Autodesk Fusion 360 part; units mm, degrees
(part 4 of 6)
sketch "Sketch5" plane through (0, 0, 0) normal (0, 1, 0) x (-1, 0, 0)
  arc A0 (-188.596, -16.7817) -> (-190.596, -18.7817) centre (-188.596, -18.7817) ccw
  line L0 (-190.596, -18.7817) -> (-190.596, -55.4069)
  line L1 (-190.596, -55.4069) -> (-190.59, -55.5639)
  line L2 (-190.59, -55.5639) -> (-190.572, -55.7209)
  line L3 (-190.572, -55.7209) -> (-190.54, -55.874)
  line L4 (-190.54, -55.874) -> (-190.499, -56.0268)
  line L5 (-190.499, -56.0268) -> (-190.444, -56.1728)
  line L6 (-190.444, -56.1728) -> (-190.379, -56.315)
  line L7 (-190.379, -56.315) -> (-190.302, -56.4526)
  line L8 (-190.302, -56.4526) -> (-190.215, -56.5838)
  line L9 (-190.215, -56.5838) -> (-190.117, -56.7062)
  line L10 (-190.117, -56.7062) -> (-190.011, -56.8219)
  line L11 (-190.011, -56.8219) -> (-189.895, -56.9281)
  line L12 (-189.895, -56.9281) -> (-189.771, -57.0258)
  line L13 (-189.771, -57.0258) -> (-189.64, -57.113)
  line L14 (-189.64, -57.113) -> (-189.504, -57.1899)
  line L15 (-189.504, -57.1899) -> (-189.362, -57.2548)
  line L16 (-189.362, -57.2548) -> (-189.214, -57.3098)
  line L17 (-189.214, -57.3098) -> (-189.063, -57.3525)
  line L18 (-189.063, -57.3525) -> (-188.908, -57.3828)
  line L19 (-188.908, -57.3828) -> (-188.753, -57.4008)
  line L20 (-188.753, -57.4008) -> (-188.597, -57.4075)
  line L21 (-188.597, -57.4075) -> (-184.1714, -57.4075)
  line L22 (-6.5216, -57.4075) -> (-2.096, -57.4075)
  line L23 (-2.096, -57.4075) -> (-1.9389, -57.4008)
  line L24 (-1.9389, -57.4008) -> (-1.7818, -57.3828)
  line L25 (-1.7818, -57.3828) -> (-1.6288, -57.3525)
  line L26 (-1.6288, -57.3525) -> (-1.4759, -57.3098)
  line L27 (-1.4759, -57.3098) -> (-1.3298, -57.2548)
  line L28 (-1.3298, -57.2548) -> (-1.1879, -57.1899)
  line L29 (-1.1879, -57.1899) -> (-1.0501, -57.113)
  line L30 (-1.0501, -57.113) -> (-0.9192, -57.0258)
  line L31 (-0.9192, -57.0258) -> (-0.7965, -56.9281)
  line L32 (-0.7965, -56.9281) -> (-0.6808, -56.8219)
  line L33 (-0.6808, -56.8219) -> (-0.5746, -56.7062)
  line L34 (-0.5746, -56.7062) -> (-0.4768, -56.5838)
  line L35 (-0.4768, -56.5838) -> (-0.39, -56.4526)
  line L36 (-0.39, -56.4526) -> (-0.3128, -56.315)
  line L37 (-0.3128, -56.315) -> (-0.248, -56.1728)
  line L38 (-0.248, -56.1728) -> (-0.1929, -56.0268)
  line L39 (-0.1929, -56.0268) -> (-0.1502, -55.874)
  line L40 (-0.1502, -55.874) -> (-0.1199, -55.7209)
  line L41 (-0.1199, -55.7209) -> (-0.102, -55.5639)
  line L42 (-0.102, -55.5639) -> (-0.0951, -55.4069)
  line L43 (-0.0951, -55.4069) -> (-0.0951, -18.7817)
  arc A1 (-0.0951, -18.7817) -> (-2.0951, -16.7817) centre (-2.0951, -18.7817) ccw
  line L44 (-2.0951, -16.7817) -> (-5.8454, -16.7817)
  arc A2 (-7.8454, -14.7817) -> (-5.8454, -16.7817) centre (-5.8454, -14.7817) ccw
  line L45 (-7.8454, -14.7817) -> (-7.8454, -2.2576)
  arc A3 (-7.8454, -2.2576) -> (-9.8454, -0.2576) centre (-9.8454, -2.2576) ccw
  line L46 (-9.8454, -0.2576) -> (-23.4739, -0.2575)
  arc A4 (-180.846, -0.2564) -> (-182.846, -2.2564) centre (-180.846, -2.2564) ccw
  line L47 (-182.846, -2.2564) -> (-182.846, -14.7817)
  arc A5 (-184.846, -16.7817) -> (-182.846, -14.7817) centre (-184.846, -14.7817) ccw
  line L48 (-184.846, -16.7817) -> (-188.596, -16.7817)
  line L49 (-31.196, -2.7823) -> (-31.196, -3.7827)
  line L50 (-31.196, -3.7827) -> (-30.3954, -3.7827)
  line L51 (-30.3954, -3.7827) -> (-30.3954, -6.8819)
  line L52 (-30.3954, -6.8819) -> (-31.196, -6.8819)
  line L53 (-31.196, -6.8819) -> (-31.196, -12.6821)
  line L54 (-31.196, -12.6821) -> (-30.3954, -12.6821)
  line L55 (-30.3954, -12.6821) -> (-30.3954, -15.7827)
  line L56 (-30.3954, -15.7827) -> (-31.196, -15.7827)
  line L57 (-31.196, -15.7827) -> (-31.196, -16.7817)
  line L58 (-31.196, -16.7817) -> (-45.1954, -16.7817)
  line L59 (-45.1954, -16.7817) -> (-45.1954, -15.7827)
  line L60 (-45.1954, -15.7827) -> (-45.9962, -15.7827)
  line L61 (-45.9962, -15.7827) -> (-45.9962, -12.6821)
  line L62 (-45.9962, -12.6821) -> (-45.1954, -12.6821)
  line L63 (-45.1954, -12.6821) -> (-45.1954, -6.8819)
  line L64 (-45.1954, -6.8819) -> (-45.9962, -6.8819)
  line L65 (-45.9962, -6.8819) -> (-45.9962, -3.7827)
  line L66 (-45.9962, -3.7827) -> (-45.1954, -3.7827)
  line L67 (-45.1954, -3.7827) -> (-45.1954, -2.7823)
  line L68 (-45.1954, -2.7823) -> (-31.196, -2.7823)
  line L69 (-159.495, -3.7827) -> (-159.495, -2.7823)
  line L70 (-159.495, -2.7823) -> (-145.496, -2.7823)
  line L71 (-145.496, -2.7823) -> (-145.496, -3.7827)
  line L72 (-145.496, -3.7827) -> (-144.695, -3.7827)
  line L73 (-144.695, -3.7827) -> (-144.695, -6.8819)
  line L74 (-144.695, -6.8819) -> (-145.496, -6.8819)
  line L75 (-145.496, -6.8819) -> (-145.496, -12.6821)
  line L76 (-145.496, -12.6821) -> (-144.695, -12.6821)
  line L77 (-144.695, -12.6821) -> (-144.695, -15.7827)
  line L78 (-144.695, -15.7827) -> (-145.496, -15.7827)
  line L79 (-145.496, -15.7827) -> (-145.496, -16.7817)
  line L80 (-145.496, -16.7817) -> (-159.495, -16.7817)
  line L81 (-159.495, -16.7817) -> (-159.495, -15.7827)
  line L82 (-159.495, -15.7827) -> (-160.296, -15.7827)
  line L83 (-160.296, -15.7827) -> (-160.296, -12.6821)
  line L84 (-160.296, -12.6821) -> (-159.495, -12.6821)
  line L85 (-159.495, -12.6821) -> (-159.495, -6.8819)
  line L86 (-159.495, -6.8819) -> (-160.296, -6.8819)
  line L87 (-160.296, -6.8819) -> (-160.296, -3.7827)
  line L88 (-160.296, -3.7827) -> (-159.495, -3.7827)
  line L89 (-59.7711, -40.8824) -> (-59.7711, -41.8828)
  line L90 (-59.7711, -41.8828) -> (-58.9703, -41.8828)
  line L91 (-58.9703, -41.8828) -> (-58.9703, -44.982)
  line L92 (-58.9703, -44.982) -> (-59.7711, -44.982)
  line L93 (-59.7711, -44.982) -> (-59.7711, -50.782)
  line L94 (-59.7711, -50.782) -> (-58.9703, -50.782)
  line L95 (-58.9703, -50.782) -> (-58.9703, -53.8826)
  line L96 (-58.9703, -53.8826) -> (-59.7711, -53.8826)
  line L97 (-59.7711, -53.8826) -> (-59.7711, -54.8816)
  line L98 (-59.7711, -54.8816) -> (-73.7704, -54.8816)
  line L99 (-73.7704, -54.8816) -> (-73.7704, -53.8826)
  line L100 (-73.7704, -53.8826) -> (-74.5712, -53.8826)
  line L101 (-74.5712, -53.8826) -> (-74.5712, -50.782)
  line L102 (-74.5712, -50.782) -> (-73.7704, -50.782)
  line L103 (-73.7704, -50.782) -> (-73.7704, -44.982)
  line L104 (-73.7704, -44.982) -> (-74.5712, -44.982)
  line L105 (-74.5712, -44.982) -> (-74.5712, -41.8828)
  line L106 (-74.5712, -41.8828) -> (-73.7704, -41.8828)
  line L107 (-73.7704, -41.8828) -> (-73.7704, -40.8824)
  line L108 (-73.7704, -40.8824) -> (-59.7711, -40.8824)
  line L109 (-92.8204, -54.8816) -> (-92.8204, -53.8826)
  line L110 (-92.8204, -53.8826) -> (-93.6198, -53.8826)
  line L111 (-93.6198, -53.8826) -> (-93.6198, -50.782)
  line L112 (-93.6198, -50.782) -> (-92.8204, -50.782)
  line L113 (-92.8204, -50.782) -> (-92.8204, -44.982)
  line L114 (-92.8204, -44.982) -> (-93.6198, -44.982)
  line L115 (-93.6198, -44.982) -> (-93.6198, -41.8828)
  line L116 (-93.6198, -41.8828) -> (-92.8204, -41.8828)
  line L117 (-92.8204, -41.8828) -> (-92.8204, -40.8824)
  line L118 (-92.8204, -40.8824) -> (-78.8211, -40.8824)
  line L119 (-78.8211, -40.8824) -> (-78.8211, -41.8828)
  line L120 (-78.8211, -41.8828) -> (-78.0203, -41.8828)
  line L121 (-78.0203, -41.8828) -> (-78.0203, -44.982)
  line L122 (-78.0203, -44.982) -> (-78.8211, -44.982)
  line L123 (-78.8211, -44.982) -> (-78.8211, -50.782)
  line L124 (-78.8211, -50.782) -> (-78.0203, -50.782)
  line L125 (-78.0203, -50.782) -> (-78.0203, -53.8826)
  line L126 (-78.0203, -53.8826) -> (-78.8211, -53.8826)
  line L127 (-78.8211, -53.8826) -> (-78.8211, -54.8816)
  line L128 (-78.8211, -54.8816) -> (-92.8204, -54.8816)
  line L129 (-16.6205, -54.8816) -> (-16.6205, -53.8826)
  line L130 (-16.6205, -53.8826) -> (-17.4212, -53.8826)
  line L131 (-17.4212, -53.8826) -> (-17.4212, -50.782)
  line L132 (-17.4212, -50.782) -> (-16.6205, -50.782)
  line L133 (-16.6205, -50.782) -> (-16.6205, -44.982)
  line L134 (-16.6205, -44.982) -> (-17.4212, -44.982)
  line L135 (-17.4212, -44.982) -> (-17.4212, -41.8828)
  line L136 (-17.4212, -41.8828) -> (-16.6205, -41.8828)
  line L137 (-16.6205, -41.8828) -> (-16.6205, -40.8824)
  line L138 (-16.6205, -40.8824) -> (-2.621, -40.8824)
  line L139 (-2.621, -40.8824) -> (-2.621, -41.8828)
  line L140 (-2.621, -41.8828) -> (-1.8204, -41.8828)
  line L141 (-1.8204, -41.8828) -> (-1.8204, -44.982)
  line L142 (-1.8204, -44.982) -> (-2.621, -44.982)
  line L143 (-2.621, -44.982) -> (-2.621, -50.782)
  line L144 (-2.621, -50.782) -> (-1.8204, -50.782)
  line L145 (-1.8204, -50.782) -> (-1.8204, -53.8826)
  line L146 (-1.8204, -53.8826) -> (-2.621, -53.8826)
  line L147 (-2.621, -53.8826) -> (-2.621, -54.8816)
  line L148 (-2.621, -54.8816) -> (-16.6205, -54.8816)
  line L149 (-174.071, -40.8824) -> (-174.071, -41.8828)
  line L150 (-174.071, -41.8828) -> (-173.27, -41.8828)
  line L151 (-173.27, -41.8828) -> (-173.27, -44.982)
  line L152 (-173.27, -44.982) -> (-174.071, -44.982)
  line L153 (-174.071, -44.982) -> (-174.071, -50.782)
  line L154 (-174.071, -50.782) -> (-173.27, -50.782)
  line L155 (-173.27, -50.782) -> (-173.27, -53.8826)
  line L156 (-173.27, -53.8826) -> (-174.071, -53.8826)
  line L157 (-174.071, -53.8826) -> (-174.071, -54.8816)
  line L158 (-174.071, -54.8816) -> (-188.07, -54.8816)
  line L159 (-188.07, -54.8816) -> (-188.07, -53.8826)
  line L160 (-188.07, -53.8826) -> (-188.871, -53.8826)
  line L161 (-188.871, -53.8826) -> (-188.871, -50.782)
  line L162 (-188.871, -50.782) -> (-188.07, -50.782)
  line L163 (-188.07, -50.782) -> (-188.07, -44.982)
  line L164 (-188.07, -44.982) -> (-188.871, -44.982)
  line L165 (-188.871, -44.982) -> (-188.871, -41.8828)
  line L166 (-188.871, -41.8828) -> (-188.07, -41.8828)
  line L167 (-188.07, -41.8828) -> (-188.07, -40.8824)
  line L168 (-188.07, -40.8824) -> (-174.071, -40.8824)
  line L169 (-126.446, -2.7823) -> (-126.446, -3.7827)
  line L170 (-126.446, -3.7827) -> (-125.645, -3.7827)
  line L171 (-125.645, -3.7827) -> (-125.645, -6.8819)
  line L172 (-125.645, -6.8819) -> (-126.446, -6.8819)
  line L173 (-126.446, -6.8819) -> (-126.446, -12.6821)
  line L174 (-126.446, -12.6821) -> (-125.645, -12.6821)
  line L175 (-125.645, -12.6821) -> (-125.645, -15.7827)
  line L176 (-125.645, -15.7827) -> (-126.446, -15.7827)
  line L177 (-126.446, -15.7827) -> (-126.446, -16.7817)
  line L178 (-126.446, -16.7817) -> (-140.445, -16.7817)
  line L179 (-140.445, -16.7817) -> (-140.445, -15.7827)
  line L180 (-140.445, -15.7827) -> (-141.246, -15.7827)
  line L181 (-141.246, -15.7827) -> (-141.246, -12.6821)
  line L182 (-141.246, -12.6821) -> (-140.445, -12.6821)
  line L183 (-140.445, -12.6821) -> (-140.445, -6.8819)
  line L184 (-140.445, -6.8819) -> (-141.246, -6.8819)
  line L185 (-141.246, -6.8819) -> (-141.246, -3.7827)
  line L186 (-141.246, -3.7827) -> (-140.445, -3.7827)
  line L187 (-140.445, -3.7827) -> (-140.445, -2.7823)
  line L188 (-140.445, -2.7823) -> (-126.446, -2.7823)
  line L189 (-26.1455, -16.7817) -> (-26.1455, -15.7827)
  line L190 (-26.1455, -15.7827) -> (-26.9462, -15.7827)
  line L191 (-26.9462, -15.7827) -> (-26.9462, -12.6821)
  line L192 (-26.9462, -12.6821) -> (-26.1455, -12.6821)
  line L193 (-26.1455, -12.6821) -> (-26.1455, -6.8819)
  line L194 (-26.1455, -6.8819) -> (-26.9462, -6.8819)
  line L195 (-26.9462, -6.8819) -> (-26.9462, -3.7827)
  line L196 (-26.9462, -3.7827) -> (-26.1455, -3.7827)
  line L197 (-26.1455, -3.7827) -> (-26.1455, -2.7823)
  line L198 (-26.1455, -2.7823) -> (-12.146, -2.7823)
  line L199 (-12.146, -2.7823) -> (-12.146, -3.7827)
  line L200 (-12.146, -3.7827) -> (-11.3454, -3.7827)
  line L201 (-11.3454, -3.7827) -> (-11.3454, -6.8819)
  line L202 (-11.3454, -6.8819) -> (-12.146, -6.8819)
  line L203 (-12.146, -6.8819) -> (-12.146, -12.6821)
  line L204 (-12.146, -12.6821) -> (-11.3454, -12.6821)
  line L205 (-11.3454, -12.6821) -> (-11.3454, -15.7827)
  line L206 (-11.3454, -15.7827) -> (-12.146, -15.7827)
  line L207 (-12.146, -15.7827) -> (-12.146, -16.7817)
  line L208 (-12.146, -16.7817) -> (-26.1455, -16.7817)
  line L209 (-64.2454, -3.7827) -> (-64.2454, -2.7823)
  line L210 (-64.2454, -2.7823) -> (-50.2461, -2.7823)
  line L211 (-50.2461, -2.7823) -> (-50.2461, -3.7827)
  line L212 (-50.2461, -3.7827) -> (-49.4453, -3.7827)
  line L213 (-49.4453, -3.7827) -> (-49.4453, -6.8819)
  line L214 (-49.4453, -6.8819) -> (-50.2461, -6.8819)
  line L215 (-50.2461, -6.8819) -> (-50.2461, -12.6821)
  line L216 (-50.2461, -12.6821) -> (-49.4453, -12.6821)
  line L217 (-49.4453, -12.6821) -> (-49.4453, -15.7827)
  line L218 (-49.4453, -15.7827) -> (-50.2461, -15.7827)
  line L219 (-50.2461, -15.7827) -> (-50.2461, -16.7817)
  line L220 (-50.2461, -16.7817) -> (-64.2454, -16.7817)
  line L221 (-64.2454, -16.7817) -> (-64.2454, -15.7827)
  line L222 (-64.2454, -15.7827) -> (-65.0462, -15.7827)
  line L223 (-65.0462, -15.7827) -> (-65.0462, -12.6821)
  line L224 (-65.0462, -12.6821) -> (-64.2454, -12.6821)
  line L225 (-64.2454, -12.6821) -> (-64.2454, -6.8819)
  line L226 (-64.2454, -6.8819) -> (-65.0462, -6.8819)
  line L227 (-65.0462, -6.8819) -> (-65.0462, -3.7827)
  line L228 (-65.0462, -3.7827) -> (-64.2454, -3.7827)
  line L229 (-135.971, -40.8824) -> (-135.971, -41.8828)
  line L230 (-135.971, -41.8828) -> (-135.17, -41.8828)
  line L231 (-135.17, -41.8828) -> (-135.17, -44.982)
  line L232 (-135.17, -44.982) -> (-135.971, -44.982)
  line L233 (-135.971, -44.982) -> (-135.971, -50.782)
  line L234 (-135.971, -50.782) -> (-135.17, -50.782)
  line L235 (-135.17, -50.782) -> (-135.17, -53.8826)
  line L236 (-135.17, -53.8826) -> (-135.971, -53.8826)
  line L237 (-135.971, -53.8826) -> (-135.971, -54.8816)
  line L238 (-135.971, -54.8816) -> (-149.97, -54.8816)
  line L239 (-149.97, -54.8816) -> (-149.97, -53.8826)
  line L240 (-149.97, -53.8826) -> (-150.771, -53.8826)
  line L241 (-150.771, -53.8826) -> (-150.771, -50.782)
  line L242 (-150.771, -50.782) -> (-149.97, -50.782)
  line L243 (-149.97, -50.782) -> (-149.97, -44.982)
  line L244 (-149.97, -44.982) -> (-150.771, -44.982)
  line L245 (-150.771, -44.982) -> (-150.771, -41.8828)
  line L246 (-150.771, -41.8828) -> (-149.97, -41.8828)
  line L247 (-149.97, -41.8828) -> (-149.97, -40.8824)
  line L248 (-149.97, -40.8824) -> (-135.971, -40.8824)
  line L249 (-73.7704, -35.8316) -> (-73.7704, -34.8327)
  line L250 (-73.7704, -34.8327) -> (-74.5712, -34.8327)
  line L251 (-74.5712, -34.8327) -> (-74.5712, -31.7321)
  line L252 (-74.5712, -31.7321) -> (-73.7704, -31.7321)
  line L253 (-73.7704, -31.7321) -> (-73.7704, -25.9319)
  line L254 (-73.7704, -25.9319) -> (-74.5712, -25.9319)
  line L255 (-74.5712, -25.9319) -> (-74.5712, -22.8327)
  line L256 (-74.5712, -22.8327) -> (-73.7704, -22.8327)
  line L257 (-73.7704, -22.8327) -> (-73.7704, -21.8323)
  line L258 (-73.7704, -21.8323) -> (-59.7711, -21.8323)
  line L259 (-59.7711, -21.8323) -> (-59.7711, -22.8327)
  line L260 (-59.7711, -22.8327) -> (-58.9703, -22.8327)
  line L261 (-58.9703, -22.8327) -> (-58.9703, -25.9319)
  line L262 (-58.9703, -25.9319) -> (-59.7711, -25.9319)
  line L263 (-59.7711, -25.9319) -> (-59.7711, -31.7321)
  line L264 (-59.7711, -31.7321) -> (-58.9703, -31.7321)
  line L265 (-58.9703, -31.7321) -> (-58.9703, -34.8327)
  line L266 (-58.9703, -34.8327) -> (-59.7711, -34.8327)
  line L267 (-59.7711, -34.8327) -> (-59.7711, -35.8316)
  line L268 (-59.7711, -35.8316) -> (-73.7704, -35.8316)
  line L269 (-54.7204, -41.8828) -> (-54.7204, -40.8824)
  line L270 (-54.7204, -40.8824) -> (-40.7211, -40.8824)
  line L271 (-40.7211, -40.8824) -> (-40.7211, -41.8828)
  line L272 (-40.7211, -41.8828) -> (-39.9203, -41.8828)
  line L273 (-39.9203, -41.8828) -> (-39.9203, -44.982)
  line L274 (-39.9203, -44.982) -> (-40.7211, -44.982)
  line L275 (-40.7211, -44.982) -> (-40.7211, -50.782)
  line L276 (-40.7211, -50.782) -> (-39.9203, -50.782)
  line L277 (-39.9203, -50.782) -> (-39.9203, -53.8826)
  line L278 (-39.9203, -53.8826) -> (-40.7211, -53.8826)
  line L279 (-40.7211, -53.8826) -> (-40.7211, -54.8816)
  line L280 (-40.7211, -54.8816) -> (-54.7204, -54.8816)
  line L281 (-54.7204, -54.8816) -> (-54.7204, -53.8826)
  line L282 (-54.7204, -53.8826) -> (-55.5212, -53.8826)
  line L283 (-55.5212, -53.8826) -> (-55.5212, -50.782)
  line L284 (-55.5212, -50.782) -> (-54.7204, -50.782)
  line L285 (-54.7204, -50.782) -> (-54.7204, -44.982)
  line L286 (-54.7204, -44.982) -> (-55.5212, -44.982)
  line L287 (-55.5212, -44.982) -> (-55.5212, -41.8828)
  line L288 (-55.5212, -41.8828) -> (-54.7204, -41.8828)
  line L289 (-130.92, -41.8828) -> (-130.92, -40.8824)
  line L290 (-130.92, -40.8824) -> (-116.92, -40.8824)
  line L291 (-116.92, -40.8824) -> (-116.92, -41.8828)
  line L292 (-116.92, -41.8828) -> (-116.119, -41.8828)
  line L293 (-116.119, -41.8828) -> (-116.119, -44.982)
  line L294 (-116.119, -44.982) -> (-116.92, -44.982)
  line L295 (-116.92, -44.982) -> (-116.92, -50.782)
  line L296 (-116.92, -50.782) -> (-116.119, -50.782)
  line L297 (-116.119, -50.782) -> (-116.119, -53.8826)
  line L298 (-116.119, -53.8826) -> (-116.92, -53.8826)
  line L299 (-116.92, -53.8826) -> (-116.92, -54.8816)
  line L300 (-116.92, -54.8816) -> (-130.92, -54.8816)
  line L301 (-130.92, -54.8816) -> (-130.92, -53.8826)
  line L302 (-130.92, -53.8826) -> (-131.721, -53.8826)
  line L303 (-131.721, -53.8826) -> (-131.721, -50.782)
  line L304 (-131.721, -50.782) -> (-130.92, -50.782)
  line L305 (-130.92, -50.782) -> (-130.92, -44.982)
  line L306 (-130.92, -44.982) -> (-131.721, -44.982)
  line L307 (-131.721, -44.982) -> (-131.721, -41.8828)
  line L308 (-131.721, -41.8828) -> (-130.92, -41.8828)
  line L309 (-21.671, -53.8826) -> (-21.671, -54.8816)
  line L310 (-21.671, -54.8816) -> (-35.6704, -54.8816)
  line L311 (-35.6704, -54.8816) -> (-35.6704, -53.8826)
  line L312 (-35.6704, -53.8826) -> (-36.4712, -53.8826)
  line L313 (-36.4712, -53.8826) -> (-36.4712, -50.782)
  line L314 (-36.4712, -50.782) -> (-35.6704, -50.782)
  line L315 (-35.6704, -50.782) -> (-35.6704, -44.982)
  line L316 (-35.6704, -44.982) -> (-36.4712, -44.982)
  line L317 (-36.4712, -44.982) -> (-36.4712, -41.8828)
  line L318 (-36.4712, -41.8828) -> (-35.6704, -41.8828)
  line L319 (-35.6704, -41.8828) -> (-35.6704, -40.8824)
  line L320 (-35.6704, -40.8824) -> (-21.671, -40.8824)
  line L321 (-21.671, -40.8824) -> (-21.671, -41.8828)
  line L322 (-21.671, -41.8828) -> (-20.8704, -41.8828)
  line L323 (-20.8704, -41.8828) -> (-20.8704, -44.982)
  line L324 (-20.8704, -44.982) -> (-21.671, -44.982)
  line L325 (-21.671, -44.982) -> (-21.671, -50.782)
  line L326 (-21.671, -50.782) -> (-20.8704, -50.782)
  line L327 (-20.8704, -50.782) -> (-20.8704, -53.8826)
  line L328 (-20.8704, -53.8826) -> (-21.671, -53.8826)
  line L329 (-97.8697, -53.8826) -> (-97.8697, -54.8816)
  line L330 (-97.8697, -54.8816) -> (-111.869, -54.8816)
  line L331 (-111.869, -54.8816) -> (-111.869, -53.8826)
  line L332 (-111.869, -53.8826) -> (-112.67, -53.8826)
  line L333 (-112.67, -53.8826) -> (-112.67, -50.782)
  line L334 (-112.67, -50.782) -> (-111.869, -50.782)
  line L335 (-111.869, -50.782) -> (-111.869, -44.982)
  line L336 (-111.869, -44.982) -> (-112.67, -44.982)
  line L337 (-112.67, -44.982) -> (-112.67, -41.8828)
  line L338 (-112.67, -41.8828) -> (-111.869, -41.8828)
  line L339 (-111.869, -41.8828) -> (-111.869, -40.8824)
  line L340 (-111.869, -40.8824) -> (-97.8697, -40.8824)
  line L341 (-97.8697, -40.8824) -> (-97.8697, -41.8828)
  line L342 (-97.8697, -41.8828) -> (-97.0703, -41.8828)
  line L343 (-97.0703, -41.8828) -> (-97.0703, -44.982)
  line L344 (-97.0703, -44.982) -> (-97.8697, -44.982)
  line L345 (-97.8697, -44.982) -> (-97.8697, -50.782)
  line L346 (-97.8697, -50.782) -> (-97.0703, -50.782)
  line L347 (-97.0703, -50.782) -> (-97.0703, -53.8826)
  line L348 (-97.0703, -53.8826) -> (-97.8697, -53.8826)
  line L349 (-155.021, -53.8826) -> (-155.021, -54.8816)
  line L350 (-155.021, -54.8816) -> (-169.02, -54.8816)
  line L351 (-169.02, -54.8816) -> (-169.02, -53.8826)
  line L352 (-169.02, -53.8826) -> (-169.821, -53.8826)
  line L353 (-169.821, -53.8826) -> (-169.821, -50.782)
  line L354 (-169.821, -50.782) -> (-169.02, -50.782)
  line L355 (-169.02, -50.782) -> (-169.02, -44.982)
  line L356 (-169.02, -44.982) -> (-169.821, -44.982)
  line L357 (-169.821, -44.982) -> (-169.821, -41.8828)
  line L358 (-169.821, -41.8828) -> (-169.02, -41.8828)
  line L359 (-169.02, -41.8828) -> (-169.02, -40.8824)
  line L360 (-169.02, -40.8824) -> (-155.021, -40.8824)
  line L361 (-155.021, -40.8824) -> (-155.021, -41.8828)
  line L362 (-155.021, -41.8828) -> (-154.22, -41.8828)
  line L363 (-154.22, -41.8828) -> (-154.22, -44.982)
  line L364 (-154.22, -44.982) -> (-155.021, -44.982)
  line L365 (-155.021, -44.982) -> (-155.021, -50.782)
  line L366 (-155.021, -50.782) -> (-154.22, -50.782)
  line L367 (-154.22, -50.782) -> (-154.22, -53.8826)
  line L368 (-154.22, -53.8826) -> (-155.021, -53.8826)
  line L369 (-111.87, -16.7817) -> (-111.87, -15.7827)
  line L370 (-111.87, -15.7827) -> (-112.671, -15.7827)
  line L371 (-112.671, -15.7827) -> (-112.671, -12.6821)
  line L372 (-112.671, -12.6821) -> (-111.87, -12.6821)
  line L373 (-111.87, -12.6821) -> (-111.87, -12.0826)
  line L374 (-111.87, -12.0826) -> (-113.396, -12.0826)
  line L375 (-113.396, -12.0826) -> (-113.396, -15.3128)
  line L376 (-113.396, -15.3128) -> (-115.12, -15.3128)
  line L377 (-115.12, -15.3128) -> (-115.12, -16.2319)
  line L378 (-115.12, -16.2319) -> (-118.42, -16.2319)
  line L379 (-118.42, -16.2319) -> (-118.42, -15.3128)
  line L380 (-118.42, -15.3128) -> (-120.146, -15.3128)
  line L381 (-120.146, -15.3128) -> (-120.146, -12.0826)
  line L382 (-120.146, -12.0826) -> (-120.971, -12.0826)
  line L383 (-120.971, -12.0826) -> (-120.971, -9.2825)
  line L384 (-120.971, -9.2825) -> (-120.146, -9.2825)
  line L385 (-120.146, -9.2825) -> (-120.146, -3.0138)
  line L386 (-120.146, -3.0138) -> (-118.42, -3.0138)
  line L387 (-118.42, -3.0138) -> (-118.42, -2.0326)
  line L388 (-118.42, -2.0326) -> (-115.12, -2.0326)
  line L389 (-115.12, -2.0326) -> (-115.12, -3.0138)
  line L390 (-115.12, -3.0138) -> (-113.396, -3.0138)
  line L391 (-113.396, -3.0138) -> (-113.396, -7.4827)
  line L392 (-113.396, -7.4827) -> (-111.87, -7.4827)
  line L393 (-111.87, -7.4827) -> (-111.87, -6.8819)
  line L394 (-111.87, -6.8819) -> (-112.671, -6.8819)
  line L395 (-112.671, -6.8819) -> (-112.671, -3.7827)
  line L396 (-112.671, -3.7827) -> (-111.87, -3.7827)
  line L397 (-111.87, -3.7827) -> (-111.87, -2.7823)
  line L398 (-111.87, -2.7823) -> (-97.8711, -2.7823)
  line L399 (-97.8711, -2.7823) -> (-97.8711, -3.7827)
  line L400 (-97.8711, -3.7827) -> (-97.0703, -3.7827)
  line L401 (-97.0703, -3.7827) -> (-97.0703, -6.8819)
  line L402 (-97.0703, -6.8819) -> (-97.8711, -6.8819)
  line L403 (-97.8711, -6.8819) -> (-97.8711, -7.4827)
  line L404 (-97.8711, -7.4827) -> (-96.3454, -7.4827)
  line L405 (-96.3454, -7.4827) -> (-96.3454, -3.0138)
  line L406 (-96.3454, -3.0138) -> (-94.6203, -3.0138)
  line L407 (-94.6203, -3.0138) -> (-94.6203, -2.0326)
  line L408 (-94.6203, -2.0326) -> (-91.3197, -2.0326)
  line L409 (-91.3197, -2.0326) -> (-91.3197, -3.0138)
  line L410 (-91.3197, -3.0138) -> (-89.596, -3.0138)
  line L411 (-89.596, -3.0138) -> (-89.596, -9.2825)
  line L412 (-89.596, -9.2825) -> (-88.7705, -9.2825)
  line L413 (-88.7705, -9.2825) -> (-88.7705, -12.0826)
  line L414 (-88.7705, -12.0826) -> (-89.596, -12.0826)
  line L415 (-89.596, -12.0826) -> (-89.596, -15.3128)
  line L416 (-89.596, -15.3128) -> (-91.3197, -15.3128)
  line L417 (-91.3197, -15.3128) -> (-91.3197, -16.2319)
  line L418 (-91.3197, -16.2319) -> (-94.6203, -16.2319)
  line L419 (-94.6203, -16.2319) -> (-94.6203, -15.3128)
  line L420 (-94.6203, -15.3128) -> (-96.3454, -15.3128)
  line L421 (-96.3454, -15.3128) -> (-96.3454, -12.0826)
  line L422 (-96.3454, -12.0826) -> (-97.8711, -12.0826)
  line L423 (-97.8711, -12.0826) -> (-97.8711, -12.6821)
  line L424 (-97.8711, -12.6821) -> (-97.0703, -12.6821)
  line L425 (-97.0703, -12.6821) -> (-97.0703, -15.7827)
  line L426 (-97.0703, -15.7827) -> (-97.8711, -15.7827)
  line L427 (-97.8711, -15.7827) -> (-97.8711, -16.7817)
  line L428 (-97.8711, -16.7817) -> (-111.87, -16.7817)
  line L429 (-69.2961, -15.7827) -> (-69.2961, -16.7817)
  line L430 (-69.2961, -16.7817) -> (-83.2954, -16.7817)
  line L431 (-83.2954, -16.7817) -> (-83.2954, -15.7827)
  line L432 (-83.2954, -15.7827) -> (-84.0962, -15.7827)
  line L433 (-84.0962, -15.7827) -> (-84.0962, -12.6821)
  line L434 (-84.0962, -12.6821) -> (-83.2954, -12.6821)
  line L435 (-83.2954, -12.6821) -> (-83.2954, -6.8819)
  line L436 (-83.2954, -6.8819) -> (-84.0962, -6.8819)
  line L437 (-84.0962, -6.8819) -> (-84.0962, -3.7827)
  line L438 (-84.0962, -3.7827) -> (-83.2954, -3.7827)
  line L439 (-83.2954, -3.7827) -> (-83.2954, -2.7823)
  line L440 (-83.2954, -2.7823) -> (-69.2961, -2.7823)
  line L441 (-69.2961, -2.7823) -> (-69.2961, -3.7827)
  line L442 (-69.2961, -3.7827) -> (-68.4953, -3.7827)
  line L443 (-68.4953, -3.7827) -> (-68.4953, -6.8819)
  line L444 (-68.4953, -6.8819) -> (-69.2961, -6.8819)
  line L445 (-69.2961, -6.8819) -> (-69.2961, -12.6821)
  line L446 (-69.2961, -12.6821) -> (-68.4953, -12.6821)
  line L447 (-68.4953, -12.6821) -> (-68.4953, -15.7827)
  line L448 (-68.4953, -15.7827) -> (-69.2961, -15.7827)
  line L449 (-40.7211, -34.8327) -> (-40.7211, -35.8316)
  line L450 (-40.7211, -35.8316) -> (-54.7204, -35.8316)
  line L451 (-54.7204, -35.8316) -> (-54.7204, -34.8327)
  line L452 (-54.7204, -34.8327) -> (-55.5212, -34.8327)
  line L453 (-55.5212, -34.8327) -> (-55.5212, -31.7321)
  line L454 (-55.5212, -31.7321) -> (-54.7204, -31.7321)
  line L455 (-54.7204, -31.7321) -> (-54.7204, -25.9319)
  line L456 (-54.7204, -25.9319) -> (-55.5212, -25.9319)
  line L457 (-55.5212, -25.9319) -> (-55.5212, -22.8327)
  line L458 (-55.5212, -22.8327) -> (-54.7204, -22.8327)
  line L459 (-54.7204, -22.8327) -> (-54.7204, -21.8323)
  line L460 (-54.7204, -21.8323) -> (-40.7211, -21.8323)
  line L461 (-40.7211, -21.8323) -> (-40.7211, -22.8327)
  line L462 (-40.7211, -22.8327) -> (-39.9203, -22.8327)
  line L463 (-39.9203, -22.8327) -> (-39.9203, -25.9319)
  line L464 (-39.9203, -25.9319) -> (-40.7211, -25.9319)
  line L465 (-40.7211, -25.9319) -> (-40.7211, -31.7321)
  line L466 (-40.7211, -31.7321) -> (-39.9203, -31.7321)
  line L467 (-39.9203, -31.7321) -> (-39.9203, -34.8327)
  line L468 (-39.9203, -34.8327) -> (-40.7211, -34.8327)
  line L469 (-111.869, -22.8327) -> (-111.869, -21.8323)
  line L470 (-111.869, -21.8323) -> (-97.8697, -21.8323)
  line L471 (-97.8697, -21.8323) -> (-97.8697, -22.8327)
  line L472 (-97.8697, -22.8327) -> (-97.0703, -22.8327)
  line L473 (-97.0703, -22.8327) -> (-97.0703, -25.9319)
  line L474 (-97.0703, -25.9319) -> (-97.8697, -25.9319)
  line L475 (-97.8697, -25.9319) -> (-97.8697, -31.7321)
  line L476 (-97.8697, -31.7321) -> (-97.0703, -31.7321)
  line L477 (-97.0703, -31.7321) -> (-97.0703, -34.8327)
  line L478 (-97.0703, -34.8327) -> (-97.8697, -34.8327)
  line L479 (-97.8697, -34.8327) -> (-97.8697, -35.8316)
  line L480 (-97.8697, -35.8316) -> (-111.869, -35.8316)
  line L481 (-111.869, -35.8316) -> (-111.869, -34.8327)
  line L482 (-111.869, -34.8327) -> (-112.67, -34.8327)
  line L483 (-112.67, -34.8327) -> (-112.67, -31.7321)
  line L484 (-112.67, -31.7321) -> (-111.869, -31.7321)
  line L485 (-111.869, -31.7321) -> (-111.869, -25.9319)
  line L486 (-111.869, -25.9319) -> (-112.67, -25.9319)
  line L487 (-112.67, -25.9319) -> (-112.67, -22.8327)
  line L488 (-112.67, -22.8327) -> (-111.869, -22.8327)
  line L489 (-92.8204, -22.8327) -> (-92.8204, -21.8323)
  line L490 (-92.8204, -21.8323) -> (-78.8211, -21.8323)
  line L491 (-78.8211, -21.8323) -> (-78.8211, -22.8327)
  line L492 (-78.8211, -22.8327) -> (-78.0203, -22.8327)
  line L493 (-78.0203, -22.8327) -> (-78.0203, -25.9319)
  line L494 (-78.0203, -25.9319) -> (-78.8211, -25.9319)
  line L495 (-78.8211, -25.9319) -> (-78.8211, -31.7321)
  line L496 (-78.8211, -31.7321) -> (-78.0203, -31.7321)
  line L497 (-78.0203, -31.7321) -> (-78.0203, -34.8327)
  line L498 (-78.0203, -34.8327) -> (-78.8211, -34.8327)
  line L499 (-78.8211, -34.8327) -> (-78.8211, -35.8316)
  line L500 (-78.8211, -35.8316) -> (-92.8204, -35.8316)
  line L501 (-92.8204, -35.8316) -> (-92.8204, -34.8327)
  line L502 (-92.8204, -34.8327) -> (-93.6198, -34.8327)
  line L503 (-93.6198, -34.8327) -> (-93.6198, -31.7321)
  line L504 (-93.6198, -31.7321) -> (-92.8204, -31.7321)
  line L505 (-92.8204, -31.7321) -> (-92.8204, -25.9319)
  line L506 (-92.8204, -25.9319) -> (-93.6198, -25.9319)
  line L507 (-93.6198, -25.9319) -> (-93.6198, -22.8327)
  line L508 (-93.6198, -22.8327) -> (-92.8204, -22.8327)
  line L509 (-35.6704, -22.8327) -> (-35.6704, -21.8323)
  line L510 (-35.6704, -21.8323) -> (-21.671, -21.8323)
  line L511 (-21.671, -21.8323) -> (-21.671, -22.8327)
  line L512 (-21.671, -22.8327) -> (-20.8704, -22.8327)
  line L513 (-20.8704, -22.8327) -> (-20.8704, -25.9319)
  line L514 (-20.8704, -25.9319) -> (-21.671, -25.9319)
  line L515 (-21.671, -25.9319) -> (-21.671, -31.7321)
  line L516 (-21.671, -31.7321) -> (-20.8704, -31.7321)
  line L517 (-20.8704, -31.7321) -> (-20.8704, -34.8327)
  line L518 (-20.8704, -34.8327) -> (-21.671, -34.8327)
  line L519 (-21.671, -34.8327) -> (-21.671, -35.8316)
  line L520 (-21.671, -35.8316) -> (-35.6704, -35.8316)
  line L521 (-35.6704, -35.8316) -> (-35.6704, -34.8327)
  line L522 (-35.6704, -34.8327) -> (-36.4712, -34.8327)
  line L523 (-36.4712, -34.8327) -> (-36.4712, -31.7321)
  line L524 (-36.4712, -31.7321) -> (-35.6704, -31.7321)
  line L525 (-35.6704, -31.7321) -> (-35.6704, -25.9319)
  line L526 (-35.6704, -25.9319) -> (-36.4712, -25.9319)
  line L527 (-36.4712, -25.9319) -> (-36.4712, -22.8327)
  line L528 (-36.4712, -22.8327) -> (-35.6704, -22.8327)
  line L529 (-16.6205, -22.8327) -> (-16.6205, -21.8323)
  line L530 (-16.6205, -21.8323) -> (-2.621, -21.8323)
  line L531 (-2.621, -21.8323) -> (-2.621, -22.8327)
  line L532 (-2.621, -22.8327) -> (-1.8204, -22.8327)
  line L533 (-1.8204, -22.8327) -> (-1.8204, -25.9319)
  line L534 (-1.8204, -25.9319) -> (-2.621, -25.9319)
  line L535 (-2.621, -25.9319) -> (-2.621, -31.7321)
  line L536 (-2.621, -31.7321) -> (-1.8204, -31.7321)
  line L537 (-1.8204, -31.7321) -> (-1.8204, -34.8327)
  line L538 (-1.8204, -34.8327) -> (-2.621, -34.8327)
  line L539 (-2.621, -34.8327) -> (-2.621, -35.8316)
  line L540 (-2.621, -35.8316) -> (-16.6205, -35.8316)
  line L541 (-16.6205, -35.8316) -> (-16.6205, -34.8327)
  line L542 (-16.6205, -34.8327) -> (-17.4212, -34.8327)
  line L543 (-17.4212, -34.8327) -> (-17.4212, -31.7321)
  line L544 (-17.4212, -31.7321) -> (-16.6205, -31.7321)
  line L545 (-16.6205, -31.7321) -> (-16.6205, -25.9319)
  line L546 (-16.6205, -25.9319) -> (-17.4212, -25.9319)
  line L547 (-17.4212, -25.9319) -> (-17.4212, -22.8327)
  line L548 (-17.4212, -22.8327) -> (-16.6205, -22.8327)
  line L549 (-164.546, -15.7827) -> (-164.546, -16.7817)
  line L550 (-164.546, -16.7817) -> (-178.545, -16.7817)
  line L551 (-178.545, -16.7817) -> (-178.545, -15.7827)
  line L552 (-178.545, -15.7827) -> (-179.346, -15.7827)
  line L553 (-179.346, -15.7827) -> (-179.346, -12.6821)
  line L554 (-179.346, -12.6821) -> (-178.545, -12.6821)
  line L555 (-178.545, -12.6821) -> (-178.545, -6.8819)
  line L556 (-178.545, -6.8819) -> (-179.346, -6.8819)
  line L557 (-179.346, -6.8819) -> (-179.346, -3.7827)
  line L558 (-179.346, -3.7827) -> (-178.545, -3.7827)
  line L559 (-178.545, -3.7827) -> (-178.545, -2.7823)
  line L560 (-178.545, -2.7823) -> (-164.546, -2.7823)
  line L561 (-164.546, -2.7823) -> (-164.546, -3.7827)
  line L562 (-164.546, -3.7827) -> (-163.745, -3.7827)
  line L563 (-163.745, -3.7827) -> (-163.745, -6.8819)
  line L564 (-163.745, -6.8819) -> (-164.546, -6.8819)
  line L565 (-164.546, -6.8819) -> (-164.546, -12.6821)
  line L566 (-164.546, -12.6821) -> (-163.745, -12.6821)
  line L567 (-163.745, -12.6821) -> (-163.745, -15.7827)
  line L568 (-163.745, -15.7827) -> (-164.546, -15.7827)
  line L569 (-116.92, -34.8327) -> (-116.92, -35.8316)
  line L570 (-116.92, -35.8316) -> (-130.92, -35.8316)
  line L571 (-130.92, -35.8316) -> (-130.92, -34.8327)
  line L572 (-130.92, -34.8327) -> (-131.721, -34.8327)
  line L573 (-131.721, -34.8327) -> (-131.721, -31.7321)
  line L574 (-131.721, -31.7321) -> (-130.92, -31.7321)
  line L575 (-130.92, -31.7321) -> (-130.92, -25.9319)
  line L576 (-130.92, -25.9319) -> (-131.721, -25.9319)
  line L577 (-131.721, -25.9319) -> (-131.721, -22.8327)
  line L578 (-131.721, -22.8327) -> (-130.92, -22.8327)
  line L579 (-130.92, -22.8327) -> (-130.92, -21.8323)
  line L580 (-130.92, -21.8323) -> (-116.92, -21.8323)
  line L581 (-116.92, -21.8323) -> (-116.92, -22.8327)
  line L582 (-116.92, -22.8327) -> (-116.119, -22.8327)
  line L583 (-116.119, -22.8327) -> (-116.119, -25.9319)
  line L584 (-116.119, -25.9319) -> (-116.92, -25.9319)
  line L585 (-116.92, -25.9319) -> (-116.92, -31.7321)
  line L586 (-116.92, -31.7321) -> (-116.119, -31.7321)
  line L587 (-116.119, -31.7321) -> (-116.119, -34.8327)
  line L588 (-116.119, -34.8327) -> (-116.92, -34.8327)
  line L589 (-155.021, -34.8327) -> (-155.021, -35.8316)
  line L590 (-155.021, -35.8316) -> (-169.02, -35.8316)
  line L591 (-169.02, -35.8316) -> (-169.02, -34.8327)
  line L592 (-169.02, -34.8327) -> (-169.821, -34.8327)
  line L593 (-169.821, -34.8327) -> (-169.821, -31.7321)
  line L594 (-169.821, -31.7321) -> (-169.02, -31.7321)
  line L595 (-169.02, -31.7321) -> (-169.02, -25.9319)
  line L596 (-169.02, -25.9319) -> (-169.821, -25.9319)
  line L597 (-169.821, -25.9319) -> (-169.821, -22.8327)
  line L598 (-169.821, -22.8327) -> (-169.02, -22.8327)
  line L599 (-169.02, -22.8327) -> (-169.02, -21.8323)
  line L600 (-169.02, -21.8323) -> (-155.021, -21.8323)
  line L601 (-155.021, -21.8323) -> (-155.021, -22.8327)
  line L602 (-155.021, -22.8327) -> (-154.22, -22.8327)
  line L603 (-154.22, -22.8327) -> (-154.22, -25.9319)
  line L604 (-154.22, -25.9319) -> (-155.021, -25.9319)
  line L605 (-155.021, -25.9319) -> (-155.021, -31.7321)
  line L606 (-155.021, -31.7321) -> (-154.22, -31.7321)
  line L607 (-154.22, -31.7321) -> (-154.22, -34.8327)
  line L608 (-154.22, -34.8327) -> (-155.021, -34.8327)
  line L609 (-135.971, -34.8327) -> (-135.971, -35.8316)
  line L610 (-135.971, -35.8316) -> (-149.97, -35.8316)
  line L611 (-149.97, -35.8316) -> (-149.97, -34.8327)
  line L612 (-149.97, -34.8327) -> (-150.771, -34.8327)
  line L613 (-150.771, -34.8327) -> (-150.771, -31.7321)
  line L614 (-150.771, -31.7321) -> (-149.97, -31.7321)
  line L615 (-149.97, -31.7321) -> (-149.97, -25.9319)
  line L616 (-149.97, -25.9319) -> (-150.771, -25.9319)
  line L617 (-150.771, -25.9319) -> (-150.771, -22.8327)
  line L618 (-150.771, -22.8327) -> (-149.97, -22.8327)
  line L619 (-149.97, -22.8327) -> (-149.97, -21.8323)
  line L620 (-149.97, -21.8323) -> (-135.971, -21.8323)
  line L621 (-135.971, -21.8323) -> (-135.971, -22.8327)
  line L622 (-135.971, -22.8327) -> (-135.17, -22.8327)
  line L623 (-135.17, -22.8327) -> (-135.17, -25.9319)
  line L624 (-135.17, -25.9319) -> (-135.971, -25.9319)
  line L625 (-135.971, -25.9319) -> (-135.971, -31.7321)
  line L626 (-135.971, -31.7321) -> (-135.17, -31.7321)
  line L627 (-135.17, -31.7321) -> (-135.17, -34.8327)
  line L628 (-135.17, -34.8327) -> (-135.971, -34.8327)
  line L629 (-188.07, -22.8327) -> (-188.07, -21.8323)
  line L630 (-188.07, -21.8323) -> (-174.071, -21.8323)
  line L631 (-174.071, -21.8323) -> (-174.071, -22.8327)
  line L632 (-174.071, -22.8327) -> (-173.27, -22.8327)
  line L633 (-173.27, -22.8327) -> (-173.27, -25.9319)
  line L634 (-173.27, -25.9319) -> (-174.071, -25.9319)
  line L635 (-174.071, -25.9319) -> (-174.071, -31.7321)
  line L636 (-174.071, -31.7321) -> (-173.27, -31.7321)
  line L637 (-173.27, -31.7321) -> (-173.27, -34.8327)
  line L638 (-173.27, -34.8327) -> (-174.071, -34.8327)
  line L639 (-174.071, -34.8327) -> (-174.071, -35.8316)
  line L640 (-174.071, -35.8316) -> (-188.07, -35.8316)
  line L641 (-188.07, -35.8316) -> (-188.07, -34.8327)
  line L642 (-188.07, -34.8327) -> (-188.871, -34.8327)
  line L643 (-188.871, -34.8327) -> (-188.871, -31.7321)
  line L644 (-188.871, -31.7321) -> (-188.07, -31.7321)
  line L645 (-188.07, -31.7321) -> (-188.07, -25.9319)
  line L646 (-188.07, -25.9319) -> (-188.871, -25.9319)
  line L647 (-188.871, -25.9319) -> (-188.871, -22.8327)
  line L648 (-188.871, -22.8327) -> (-188.07, -22.8327)
  line L649 (-118.42, -2.0326) -> (-120.971, -2.0326)
  line L650 (-120.971, -2.0326) -> (-120.971, -12.0826)
  line L651 (-88.7705, -16.7817) -> (-120.971, -16.7817)
  line L652 (-120.971, -16.7817) -> (-120.971, -2.0326)
  line L653 (-120.971, -2.0326) -> (-88.7705, -2.0326)
  line L654 (-88.7705, -2.0326) -> (-88.7705, -16.7817)
  spline S0 degree 2 poles (-184.1714, -57.4075) (-176.3801, -57.4075) (-176.3801, -64.9763) knots 0 0 0 1 1 1
  arc A6 (-176.3801, -64.9763) -> (-162.7837, -64.9763) centre (-169.5819, -64.5335) ccw
  spline S1 degree 2 poles (-154.9924, -57.4075) (-162.7837, -57.4075) (-162.7837, -64.9763) knots 0 0 0 1 1 1
  line L655 (-154.9924, -57.4075) -> (-35.7006, -57.4075)
  spline S2 degree 2 poles (-35.7006, -57.4075) (-27.9093, -57.4075) (-27.9093, -64.9763) knots 0 0 0 1 1 1
  arc A7 (-27.9093, -64.9763) -> (-14.3129, -64.9763) centre (-21.1111, -64.5335) ccw
  spline S3 degree 2 poles (-6.5216, -57.4075) (-14.3129, -57.4075) (-14.3129, -64.9763) knots 0 0 0 1 1 1
  line L656 (-167.2132, -68.8727) -> (-171.8315, -68.9414)
  line L657 (-171.8315, -68.9414) -> (-174.2002, -64.9763)
  line L658 (-174.2002, -64.9763) -> (-171.9506, -60.9423)
  line L659 (-171.9506, -60.9423) -> (-167.3323, -60.8736)
  line L660 (-167.3323, -60.8736) -> (-164.9636, -64.8387)
  line L661 (-164.9636, -64.8387) -> (-167.2132, -68.8727)
  line L662 (-18.8615, -68.9414) -> (-23.4798, -68.8727)
  line L663 (-23.4798, -68.8727) -> (-25.7294, -64.8387)
  line L664 (-25.7294, -64.8387) -> (-23.3607, -60.8736)
  line L665 (-23.3607, -60.8736) -> (-18.7424, -60.9423)
  line L666 (-18.7424, -60.9423) -> (-16.4928, -64.9763)
  line L667 (-16.4928, -64.9763) -> (-18.8615, -68.9414)
  spline S4 degree 2 poles (-23.4739, -0.2575) (-31.3819, -0.2565) (-31.3817, 7.3119) knots 0 0 0 1 1 1
  arc A8 (-31.3817, 7.3119) -> (-44.977, 7.3123) centre (-38.1793, 6.8699) ccw
  spline S5 degree 2 poles (-52.8852, -0.2567) (-44.9772, -0.2561) (-44.977, 7.3123) knots 0 0 0 1 1 1
  line L668 (-52.8852, -0.2567) -> (-52.887, -0.2573)
  line L669 (-52.887, -0.2573) -> (-137.8078, -0.2567)
  spline S6 degree 2 poles (-137.8078, -0.2567) (-145.7158, -0.2561) (-145.716, 7.3123) knots 0 0 0 1 1 1
  arc A9 (-145.716, 7.3123) -> (-159.3113, 7.3119) centre (-152.5137, 6.8699) ccw
  spline S7 degree 2 poles (-167.0351, -0.2565) (-159.3111, -0.1679) (-159.3113, 7.3119) knots 0.011703 0.011703 0.011703 1 1 1
  line L670 (-167.0351, -0.2565) -> (-180.846, -0.2564)
  line L671 (-35.9298, 3.2095) -> (-40.548, 3.2783)
  line L672 (-40.548, 3.2783) -> (-42.7976, 7.3122)
  line L673 (-42.7976, 7.3122) -> (-40.4289, 11.2774)
  line L674 (-40.4289, 11.2774) -> (-35.8106, 11.2086)
  line L675 (-35.8106, 11.2086) -> (-33.561, 7.1747)
  line L676 (-33.561, 7.1747) -> (-35.9298, 3.2095)
  line L677 (-154.7632, 3.2095) -> (-157.132, 7.1747)
  line L678 (-157.132, 7.1747) -> (-154.8824, 11.2086)
  line L679 (-154.8824, 11.2086) -> (-150.2641, 11.2774)
  line L680 (-150.2641, 11.2774) -> (-147.8954, 7.3122)
  line L681 (-147.8954, 7.3122) -> (-150.145, 3.2783)
  line L682 (-150.145, 3.2783) -> (-154.7632, 3.2095)
  point P0 (-88.7705, -16.7817)
  constraint horizontal L649
  constraint vertical L650
  constraint coincident L387.end L388.start
  constraint coincident L382.end L383.start
  constraint horizontal L651
  constraint vertical L652
  constraint horizontal L653
  constraint vertical L654
  constraint coincident P0 L651.start
extrude "Extrude7" cut sketch "Sketch5" against normal blind 5 contours L369 L370 L371 L372 L373 L374 L375 L376 L377 L378 L379 L380 L381 L382 L651 L652 | L369 L370 L371 L372 L373 L374 L375 L376 L377 L378 L379 L380 L381 L382 L383 L384 L385 L386 L387 L388 L389 L390 L391 L392 L393 L394 L395 L396 L397 L398 L399 L400 L401 L402 L403 L404 L405 L406 L407 L408 L409 L410 L411 L412 L413 L414 L415 L416 L417 L418 L419 L420 L421 L422 L423 L424 L425 L426 L427 L428 L650 L651 L652 L653 L654 | L414 L415 L416 L417 L418 L419 L420 L421 L422 L423 L424 L425 L426 L427 L651 L654 | L384 L385 L386 L387 L649 L650 L652 L653 | L409 L410 L411 L412 L653 L654 | L389 L390 L391 L392 L393 L394 L395 L396 L397 L398 L399 L400 L401 L402 L403 L404 L405 L406 L407 L653